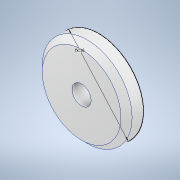
# Autodesk Inventor part: Capstondisc_v2_Anschlagscheibe
Saved by Autodesk Inventor 2022 (Build 260153000, 153)
## iProperties
Created: 2022-08-01
Part Number: Capstondisc_v2_Anschlagscheibe
Material: Aluminium 6061
Document SubType Name: Modeling
Designer: alexw
Density: 2.7 g/cm^3
Appearance: Aluminium - flach
Mass: 1.49003 g
Surface Area: 5.3606 cm^2
Volume: 0.551863 cm^3
Author: alexw
Autodesk Inventor part; units mm, degrees
ref_plane "YZ Plane" through (0, 0, 0) normal (1, 0, 0) x (0, 1, 0)
ref_plane "XZ Plane" through (0, 0, 0) normal (0, 1, 0) x (-1, 0, 0)
ref_plane "XY Plane" through (0, 0, 0) normal (0, 0, 1) x (1, 0, 0)
sketch "Skizze1" plane through (0, 0, 0) normal (0, 0, 1) x (1, 0, 0)
  circle A0 centre (0, 0) radius 8
  dimension "d0" = 16
  constraints: 2 coincident, 1 centre point
  measures "d0" diameter of A0
extrude "Extrusion1" add sketch "Skizze1" along normal blind 3
chamfer "Fase1" distance 1 angle 45 1 edges at (-8, 0, 3)
hole "Bohrung1" at (0, 0, 0) direction (0, 0, 1) diameter 3.4 depth 8 tip angle 118 clearance for "Sechskantkopfschraube DIN EN 24017" size "M3" standard "DIN"
